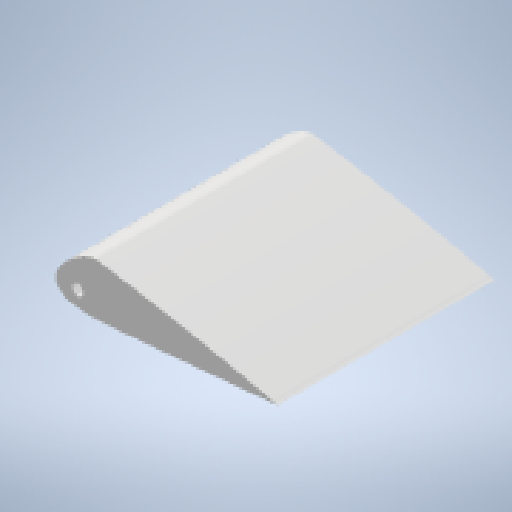
# Autodesk Inventor part: 4P.01.01.01-TW-v1-Flap Shape Definition
Saved by Autodesk Inventor 2025.2 (Build 292293000, 293)
## iProperties
Created: 2024-11-18
Part Number: 4P.01.01.01-TW-v1-Flap Shape Definition
Material: Generic
Document SubType Name: Modeling
Designer: thoma
Density: 1 g/cm^3
Appearance: Default
Author: thoma
Autodesk Inventor part; units mm, degrees
ref_plane "YZ Plane" through (0, 0, 0) normal (1, 0, 0) x (0, 1, 0)
ref_plane "XZ Plane" through (0, 0, 0) normal (0, 1, 0) x (-1, 0, 0)
ref_plane "XY Plane" through (0, 0, 0) normal (0, 0, 1) x (1, 0, 0)
sketch "Sketch1" plane through (0, 0, 0) normal (0, 0, 1) x (1, 0, 0)
  spline S0 degree 5 poles (300, 0) (300.0016, 0.0244) (299.7036, 0.09) (298.2843, 0.2856) (298.1861, 0.6201) (294.2411, 1.1852) (292.5088, 1.8941) (287.5168, 2.8048) (283.3251, 3.8823) (277.2635, 5.114) (271.0288, 6.4738) (263.7046, 7.9415) (255.8588, 9.4927) (247.2609, 11.1039) (238.105, 12.7506) (228.3746, 14.4096) (218.1643, 16.0564) (207.5185, 17.6669) (196.5111, 19.219) (185.2054, 20.6879) (173.6732, 22.052) (161.9834, 23.2887) (150.21, 24.3752) (138.4162, 25.2964) (126.6928, 26.0196) (115.0744, 26.5602) (103.5988, 26.7997) (92.4288, 26.7578) (81.6023, 26.4231) (71.2108, 25.8005) (61.3178, 24.8978) (51.9933, 23.7307) (43.2967, 22.3175) (35.2844, 20.6817) (28.0043, 18.8519) (21.5007, 16.8582) (15.8056, 14.7303) (10.9426, 12.4987) (6.9231, 10.1816) (3.745, 7.791) (1.4298, 5.3026) (0.027, 2.7048) (-0.2762, -0.026) (0.5609, -2.6395) (2.4314, -4.909) (5.1526, -6.9052) (8.674, -8.6574) (12.9744, -10.2099) (18.0511, -11.5643) (23.8856, -12.7277) (30.4535, -13.6933) (37.7169, -14.4652) (45.6371, -15.0404) (54.1678, -15.428) (63.2602, -15.6353) (72.8628, -15.6753) (82.9246, -15.5641) (93.3855, -15.3196) (104.2036, -14.9665) (115.2834, -14.5145) (126.6481, -14.0171) (138.1928, -13.3887) (149.8108, -12.6841) (161.4481, -11.9059) (173.0242, -11.0809) (184.4692, -10.2189) (195.7125, -9.3406) (206.6821, -8.4534) (217.315, -7.5734) (227.5362, -6.706) (237.2988, -5.8637) (246.5067, -5.0508) (255.1715, -4.2808) (263.0989, -3.5455) (270.5088, -2.8843) (276.8391, -2.2398) (282.9867, -1.7375) (287.2724, -1.1764) (292.3303, -0.9034) (294.139, -0.4203) (298.1203, -0.3746) (298.262, -0.0558) (299.6943, -0.05) (299.9984, -0.0244) (300, 0) knots 0 0 0 0 0 0 0.005555 0.010406 0.017155 0.025351 0.034694 0.045016 0.056192 0.068127 0.080735 0.093944 0.107687 0.121902 0.13653 0.151515 0.166802 0.182339 0.198074 0.213956 0.229934 0.245959 0.261986 0.277975 0.293876 0.30964 0.325217 0.340551 0.355583 0.370262 0.384536 0.398352 0.411658 0.424397 0.436516 0.447959 0.458676 0.468629 0.477816 0.486311 0.494269 0.501928 0.509582 0.517526 0.525994 0.535136 0.54502 0.555644 0.566968 0.578942 0.591513 0.604627 0.618231 0.632275 0.64671 0.661487 0.676558 0.691886 0.707429 0.72314 0.738971 0.754875 0.770794 0.786673 0.802462 0.818112 0.833572 0.848791 0.863714 0.878289 0.892459 0.906165 0.919343 0.931928 0.943844 0.955007 0.965319 0.974656 0.982848 0.989595 0.994445 1 1 1 1 1 1
  line L0 (200, 103) -> (200, -97) construction
  line L1 (0, -164.4758) -> (0, 307.8549) construction
  line L2 (210, 0) -> (210, -12) construction
  line L3 (210, 0) -> (222, 0) construction
  spline S1 degree 4 poles (218.5257, 15.9738) (209.601, 17.344) (179.4452, -9.5392) (209.7943, -8.4144) (227.9538, -6.6666) knots 0 0 0 0 0 1 1 1 1 1
  line L4 (221.1774, 15.5667) -> (215.874, 16.3809) construction
  arc A0 (220.2542, 15.1852) -> (216.6402, 15.74) centre (217.9961, 12.5243) ccw construction
  line L5 (222.2571, -7.2149) -> (233.6505, -6.1183) construction
  arc A1 (223.3931, -7.0631) -> (232.5064, -6.186) centre (204.1762, 240.3791) ccw construction
  circle A2 centre (210, 0) radius 2.5
  point P0 (0, 0)
  point P1 (298.1739, 0.4338)
  point P2 (295.9008, 0.9681)
  point P3 (292.7367, 1.7025)
  point P4 (288.6996, 2.6229)
  point P5 (283.8129, 3.7134)
  point P6 (278.1048, 4.9545)
  point P7 (271.6086, 6.3255)
  point P8 (264.3621, 7.8039)
  point P9 (256.4085, 9.3663)
  point P10 (247.7946, 10.9887)
  point P11 (238.572, 12.6468)
  point P12 (228.7959, 14.3166)
  point P13 (207.8235, 17.5944)
  point P14 (196.755, 19.155)
  point P15 (185.388, 20.6319)
  point P16 (173.7924, 22.0023)
  point P17 (162.0405, 23.2434)
  point P18 (150.2055, 24.3336)
  point P19 (138.3615, 25.2522)
  point P20 (126.5832, 25.98)
  point P21 (114.8976, 26.493)
  point P22 (103.3635, 26.7315)
  point P23 (92.1183, 26.6775)
  point P24 (81.2367, 26.3292)
  point P25 (70.7922, 25.689)
  point P26 (60.8541, 24.7656)
  point P27 (51.489, 23.5734)
  point P28 (42.7587, 22.131)
  point P29 (34.7199, 20.4618)
  point P30 (27.4239, 18.5934)
  point P31 (20.9172, 16.5555)
  point P32 (15.2385, 14.379)
  point P33 (10.422, 12.0954)
  point P34 (6.4944, 9.7347)
  point P35 (3.4767, 7.3239)
  point P36 (1.3836, 4.8867)
  point P37 (0.2238, 2.4411)
  point P38 (0, 0)
  point P39 (0.7011, -2.3487)
  point P40 (2.31, -4.5201)
  point P41 (4.8123, -6.5094)
  point P42 (8.1885, -8.3112)
  point P43 (12.414, -9.9204)
  point P44 (17.4594, -11.3319)
  point P45 (23.2908, -12.5418)
  point P46 (29.871, -13.5477)
  point P47 (37.1583, -14.3505)
  point P48 (45.1092, -14.9526)
  point P49 (53.6766, -15.3609)
  point P50 (62.8101, -15.5853)
  point P51 (72.4581, -15.639)
  point P52 (82.566, -15.5385)
  point P53 (93.0768, -15.3033)
  point P54 (103.9314, -14.9544)
  point P55 (115.0689, -14.514)
  point P56 (126.4866, -13.9956)
  point P57 (138.1008, -13.3755)
  point P58 (149.7945, -12.6672)
  point P59 (161.4972, -11.8896)
  point P60 (173.1378, -11.061)
  point P61 (184.6455, -10.1973)
  point P62 (195.9501, -9.3141)
  point P63 (206.9814, -8.4237)
  point P64 (217.6716, -7.5381)
  point P65 (227.9538, -6.6666)
  point P66 (237.7638, -5.8185)
  point P67 (247.0398, -5.0019)
  point P68 (255.7236, -4.2234)
  point P69 (263.7597, -3.4905)
  point P70 (271.0965, -2.8098)
  point P71 (277.6872, -2.1882)
  point P72 (283.4889, -1.6323)
  point P73 (288.4641, -1.1487)
  point P74 (292.5804, -0.7434)
  point P75 (295.8102, -0.4221)
  point P76 (298.1328, -0.1887)
  point P77 (299.5323, -0.0474)
  point P78 (200, 0)
  point P79 (223.7705, -7.0234)
  dimension "d0" = 200
  dimension "d2" = 200
  dimension "d3" = 12
  dimension "d4" = 90
  dimension "d5" = 10
  dimension "d17" = 5
  constraints: 10 end point, 4 midpoint, 3 centre point, 2 coincident, 2 point on circle, 2 vertical, 1 horizontal, 1 perpendicular, 1 point on line, 88 other
  measures "d0" distance of L0.start L0.end
  measures "d2" distance between parallel lines of L1 L0
  measures "d3" distance of L2.start L2.end
  measures "d4" angle of L2 L3
  measures "d5" distance between parallel lines of L0 L2
  measures "d17" diameter of A2
extrude "Extrusion2" add sketch "Sketch1" along normal blind 97.75 contours S0 S1 picked at (264.3061, 0.3433)
body "Solid2"
